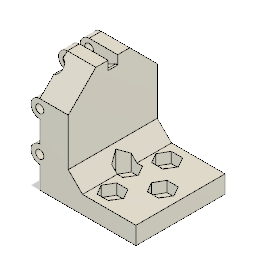
Anclaje base (Autodesk Fusion 360 design; units mm, degrees)
Autodesk Fusion 360 part; units mm, degrees
ref_plane "PlanoDeObra1" through (20, 0, 0) normal (1, 0, 0) x (0, 1, 0)
sketch "Boceto3" plane through (20, 0, 0) normal (1, 0, 0) x (0, 0, -1)
  line L0 (-0.475, 13.25) -> (-25.475, 13.25)
  line L1 (-25.475, 13.25) -> (-25.475, -16.75)
  line L2 (-25.475, -16.75) -> (-0.475, -16.75)
  line L3 (-0.475, -16.75) -> (-0.475, 13.25)
  line L4 (-25.475, -11.75) -> (-0.475, -11.75)
  line L5 (-17.2083, -5.5132) -> (-8.7417, -5.5132)
  line L6 (-8.7417, -5.5132) -> (-8.7417, -10.5132)
  line L7 (-8.7417, -10.5132) -> (-17.2083, -10.5132)
  line L8 (-17.2083, -10.5132) -> (-17.2083, -5.5132)
  line L9 (-3.9417, -5.5132) -> (-0.475, -5.5132)
  line L10 (-0.475, -5.5132) -> (-0.475, -10.5132)
  line L11 (-0.475, -10.5132) -> (-3.9417, -10.5132)
  line L12 (-3.9417, -10.5132) -> (-3.9417, -5.5132)
  line L13 (-22.0083, -5.5132) -> (-25.475, -5.5132)
  line L14 (-25.475, -5.5132) -> (-25.475, -10.5132)
  line L15 (-25.475, -10.5132) -> (-22.0083, -10.5132)
  line L16 (-22.0083, -10.5132) -> (-22.0083, -5.5132)
  line L17 (-19.5083, -9.4526) -> (-17.2083, -9.4526) construction
  line L18 (-8.7417, -8.7956) -> (-6.4417, -8.7956) construction
  line L19 (-22.0083, -5.5132) -> (-17.2083, -5.5132)
  line L20 (-17.2083, -10.5132) -> (-22.0083, -10.5132)
  line L21 (-8.7417, -5.5132) -> (-3.9417, -5.5132)
  line L22 (-3.9417, -10.5132) -> (-8.7417, -10.5132)
  line L23 (-0.475, -8.0132) -> (-25.475, -8.0132)
  line L24 (-25.475, 5.5132) -> (-22.0083, 5.5132)
  line L25 (-22.0083, 5.5132) -> (-22.0083, 0.5132)
  line L26 (-22.0083, 0.5132) -> (-25.475, 0.5132)
  line L27 (-25.475, 0.5132) -> (-25.475, 5.5132)
  line L28 (-3.9417, 5.5132) -> (-0.475, 5.5132)
  line L29 (-0.475, 5.5132) -> (-0.475, 0.5132)
  line L30 (-0.475, 0.5132) -> (-3.9417, 0.5132)
  line L31 (-3.9417, 0.5132) -> (-3.9417, 5.5132)
  line L32 (-22.0083, 5.5132) -> (-17.2083, 5.5132)
  line L33 (-17.2083, 5.5132) -> (-17.2083, 0.5132)
  line L34 (-17.2083, 0.5132) -> (-22.0083, 0.5132)
  line L35 (-3.9417, 5.5132) -> (-8.7417, 5.5132)
  line L36 (-8.7417, 5.5132) -> (-8.7417, 0.5132)
  line L37 (-8.7417, 0.5132) -> (-3.9417, 0.5132)
  line L38 (-25.475, 3.0132) -> (-0.475, 3.0132)
  line L39 (-17.7382, 13.25) -> (-25.475, 5.5132)
  line L40 (-8.2118, 13.25) -> (-0.475, 5.5132)
  line L41 (-19.5083, -5.5132) -> (-22.975, -5.5132) construction
  line L42 (-22.975, -10.5132) -> (-22.975, -5.5132) construction
  line L43 (-22.975, -10.5132) -> (-19.5083, -10.5132) construction
  line L44 (-19.5083, -10.5132) -> (-19.5083, -5.5132) construction
  line L45 (-2.975, -5.5132) -> (-6.4417, -5.5132) construction
  line L46 (-6.4417, -10.5132) -> (-6.4417, -5.5132) construction
  line L47 (-6.4417, -10.5132) -> (-2.975, -10.5132) construction
  line L48 (-2.975, -10.5132) -> (-2.975, -5.5132) construction
  line L49 (-2.975, 10.5132) -> (-6.4417, 10.5132) construction
  line L50 (-6.4417, 5.5132) -> (-6.4417, 10.5132) construction
  line L51 (-6.4417, 5.5132) -> (-2.975, 5.5132) construction
  line L52 (-2.975, 5.5132) -> (-2.975, 10.5132) construction
  line L53 (-19.5083, 10.5132) -> (-22.975, 10.5132) construction
  line L54 (-22.975, 5.5132) -> (-22.975, 10.5132) construction
  line L55 (-22.975, 5.5132) -> (-19.5083, 5.5132) construction
  line L56 (-19.5083, 5.5132) -> (-19.5083, 10.5132) construction
  line L57 (-11.2417, 10.5132) -> (-14.7083, 10.5132) construction
  line L58 (-14.7083, 5.5132) -> (-14.7083, 10.5132) construction
  line L59 (-14.7083, 5.5132) -> (-11.2417, 5.5132) construction
  line L60 (-11.2417, 5.5132) -> (-11.2417, 10.5132) construction
  line L61 (-14.7083, 5.5132) -> (-19.5083, 5.5132) construction
  line L62 (-6.4417, 5.5132) -> (-11.2417, 5.5132) construction
  line L63 (-22.0083, 0.5132) -> (-22.0083, -1.2368)
  line L64 (-22.0083, -1.2368) -> (-17.2083, -1.2368)
  line L65 (-17.2083, -1.2368) -> (-17.2083, 0.5132)
  line L66 (-8.7417, 0.5132) -> (-8.7417, -1.2368)
  line L67 (-8.7417, -1.2368) -> (-3.9417, -1.2368)
  line L68 (-3.9417, -1.2368) -> (-3.9417, 0.5132)
  line L69 (-22.0083, -5.5132) -> (-22.0083, -3.7632)
  line L70 (-22.0083, -3.7632) -> (-17.2083, -3.7632)
  line L71 (-17.2083, -3.7632) -> (-17.2083, -5.5132)
  line L72 (-3.9417, -5.5132) -> (-3.9417, -3.7632)
  line L73 (-3.9417, -3.7632) -> (-8.7417, -3.7632)
  line L74 (-8.7417, -3.7632) -> (-8.7417, -5.5132)
  line L75 (-8.7417, 0.5132) -> (-17.2083, 0.5132)
  line L76 (-17.2083, 5.5132) -> (-8.7417, 5.5132)
  line L77 (-8.2118, 13.25) -> (-8.2118, 8.25)
  line L78 (-8.2118, 8.25) -> (-17.7382, 8.25)
  line L79 (-17.7382, 8.25) -> (-17.7382, 13.25)
  line L80 (-8.2118, 10.75) -> (-17.7382, 10.75)
  line L81 (-14.325, 13.25) -> (-14.325, 8.25)
  line L82 (-11.625, 8.25) -> (-11.625, 13.25)
  line L83 (-11.625, 11.8923) -> (-8.2118, 11.8923) construction
  line L84 (-14.325, 11.8923) -> (-17.7382, 11.8923) construction
  line L85 (-11.625, 8.25) -> (-11.625, 7.5)
  line L86 (-11.625, 7.5) -> (-14.325, 7.5)
  line L87 (-14.325, 7.5) -> (-14.325, 8.25)
  line L88 (-17.2083, 5.0132) -> (-8.7417, 5.0132)
  line L89 (-17.2083, -3.7632) -> (-17.2083, -3.3632)
  line L90 (-17.2083, -3.3632) -> (-22.0083, -3.3632)
  line L91 (-22.0083, -3.3632) -> (-22.0083, -3.7632)
  line L92 (-3.9417, -3.7632) -> (-3.9417, -3.3632)
  line L93 (-3.9417, -3.3632) -> (-8.7417, -3.3632)
  line L94 (-8.7417, -3.3632) -> (-8.7417, -3.7632)
  line L95 (-3.9417, -1.2368) -> (-3.9417, -1.6368)
  line L96 (-3.9417, -1.6368) -> (-8.7417, -1.6368)
  line L97 (-8.7417, -1.6368) -> (-8.7417, -1.2368)
  line L98 (-17.2083, -1.2368) -> (-17.2083, -1.6368)
  line L99 (-17.2083, -1.6368) -> (-22.0083, -1.6368)
  line L100 (-22.0083, -1.6368) -> (-22.0083, -1.2368)
  line L101 (-8.7417, -6.0132) -> (-17.2083, -6.0132)
  dimension "d7" = 12
  dimension "d15" = 30
  dimension "d16" = 25
  dimension "d17" = 5
  dimension "d97" = 0.4
  dimension "d107" = 4.8
  dimension "d108" = 4.8
  dimension "d112" = 45
  dimension "d113" = 45
  dimension "d114" = 2.7
  dimension "d131" = 3.25
  dimension "d166" = 0.5
  dimension "d179" = 0.4
  dimension "d180" = 4.25
  dimension "d181" = 0.4
  dimension "d182" = 4.25
  dimension "d183" = 0.4
  dimension "d184" = 0.4
  dimension "d185" = 4.25
  dimension "d186" = 4.25
  dimension "d187" = 0.5
  constraint vertical L1
  constraint horizontal L2
  constraint vertical L3
  constraint coincident L1 L4.start
  constraint coincident L3 L4.end
  constraint perpendicular L3 L4
  constraint horizontal L5
  constraint vertical L6
  constraint horizontal L7
  constraint vertical L8
  constraint horizontal L9
  constraint vertical L10
  constraint horizontal L11
  constraint vertical L12
  constraint horizontal L13
  constraint vertical L14
  constraint horizontal L15
  constraint vertical L16
  constraint collinear L5 L13
  constraint collinear L5 L9
  constraint collinear L1 L14
  constraint collinear L3 L10
  constraint equal L17 L18
  constraint midpoint L10 L23.start
  constraint midpoint L14 L23.end
  constraint horizontal L24
  constraint vertical L25
  constraint horizontal L26
  constraint vertical L27
  constraint horizontal L28
  constraint vertical L29
  constraint horizontal L30
  constraint vertical L31
  constraint collinear L26 L30
  constraint collinear L1 L27
  constraint collinear L3 L29
  constraint horizontal L32
  constraint vertical L33
  constraint horizontal L34
  constraint horizontal L35
  constraint vertical L36
  constraint horizontal L37
  constraint midpoint L27 L38.start
  constraint midpoint L29 L38.end
  constraint coincident L0 L39.start
  constraint coincident L0 L40.start
  constraint equal L15 L43
  constraint equal L11 L47
  constraint equal L8 L44
  constraint equal L16 L44
  constraint coincident L8 L17.end
  constraint coincident L17.start L44
  constraint perpendicular L17 L44
  constraint coincident L6 L18.start
  constraint coincident L18.end L46
  constraint equal L12 L46
  constraint collinear L7 L47
  constraint equal L31 L50
  constraint equal L25 L56
  constraint coincident L30.end L31.start
  constraint coincident L25.end L26.start
  constraint equal L28 L49
  constraint equal L24 L53
  constraint collinear L28 L59
  constraint equal L34 L61
  constraint equal L37 L62
  constraint perpendicular L34 L63
  constraint perpendicular L25 L64
  constraint perpendicular L37 L66
  constraint perpendicular L36 L67
  constraint perpendicular L67 L68
  constraint perpendicular L64 L65
  constraint perpendicular L13 L69
  constraint perpendicular L16 L70
  constraint perpendicular L21 L72
  constraint perpendicular L72 L73
  constraint perpendicular L73 L74
  constraint perpendicular L70 L71
  constraint perpendicular L18 L46
  constraint perpendicular L0 L77
  constraint perpendicular L77 L78
  constraint perpendicular L78 L79
  constraint equal L58 L79
  constraint midpoint L77 L80.start
  constraint midpoint L79 L80.end
  constraint parallel L79 L81
  constraint parallel L77 L82
  constraint coincident L82 L83.start
  constraint coincident L77 L83.end
  constraint perpendicular L77 L83
  constraint coincident L81 L84.start
  constraint coincident L79 L84.end
  constraint perpendicular L79 L84
  constraint equal L83 L84
  constraint perpendicular L78 L85
  constraint perpendicular L78 L87
  constraint parallel L78 L86
  constraint coincident L33 L88.start
  constraint coincident L36 L88.end
  constraint perpendicular L36 L88
  constraint perpendicular L70 L89
  constraint perpendicular L71 L90
  constraint perpendicular L90 L91
  constraint perpendicular L73 L92
  constraint perpendicular L72 L93
  constraint perpendicular L93 L94
  constraint perpendicular L67 L95
  constraint perpendicular L95 L96
  constraint perpendicular L96 L97
  constraint perpendicular L64 L98
  constraint perpendicular L65 L99
  constraint perpendicular L99 L100
  constraint coincident L6 L101.start
  constraint coincident L8 L101.end
  constraint perpendicular L8 L101
  measures "d15" distance of L0.end L1.end
  measures "d16" distance of L1.end L2.end
  measures "d17" distance of L2 L4
  measures "d107" distance of L6 L12
  measures "d108" distance of L31 L36
  measures "d112" angle of L28.end L40.start L50.start
  measures "d113" angle of L24.start L39.start L55.end
  measures "d114" distance of L81 L82
  measures "d131" distance of L80 L86
  measures "d166" distance of L76 L88
  measures "d179" distance of L70 L90
  measures "d180" distance of L23 L70
  measures "d181" distance of L73 L93
  measures "d182" distance of L23 L73
  measures "d183" distance of L67 L96
  measures "d184" distance of L64 L99
  measures "d185" distance of L38 L64
  measures "d186" distance of L38 L67
  measures "d187" distance of L5 L101
extrude "Extruir5" add sketch "Boceto3" along normal blind 8 contours L0 L77 L80 L82 | L24 L28 L32 L35 L39 L40 L76 L77 L78 L79 L85 L86 L87 | L3 L28 L29 L31 L38 | L0 L80 L81 L82 | L77 L78 L80 L82 | L3 L29 L30 L31 L38 | L31 L35 L36 L38 | L0 L79 L80 L81 | L78 L80 L81 L82 | L1 L3 L5 L9 L13 L26 L30 L63 L65 L66 L68 L69 L71 L72 L74 L75 L89 L90 L91 L92 L93 L94 L95 L96 L97 L98 L99 L100 | L31 L36 L37 L38 | L33 L36 L76 L88 | L78 L79 L80 L81 | L78 L85 L86 L87 | L3 L9 L10 L12 L23 | L37 L66 L67 L68 | L33 L36 L38 L88 | L33 L36 L38 L75 | L25 L32 L33 L38 | L1 L24 L25 L27 L38 | L3 L10 L11 L12 L23 | L6 L12 L21 L23 | L21 L72 L73 L74 | L67 L95 L96 L97 | L25 L33 L34 L38 | L1 L25 L26 L27 L38 | L1 L3 L4 L7 L11 L15 L20 L22 | L6 L12 L22 L23 | L5 L6 L8 L101 | L73 L92 L93 L94 | L34 L63 L64 L65 | L1 L2 L3 L4 | L6 L8 L23 L101 | L6 L7 L8 L23 | L8 L16 L19 L23 | L19 L69 L70 L71 | L64 L98 L99 L100 | L1 L13 L14 L16 L23 | L8 L16 L20 L23 | L70 L89 L90 L91 | L1 L14 L15 L16 L23
extrude "Extruir6" add sketch "Boceto3" along normal blind 27 contours L1 L2 L3 L4
revolve "Revolución13" add sketch "Boceto3" angle 360 about axis through (20, -8.0132, 0.475) along (0, 0, 1) contours L3 L9 L10 L12 L23 | L6 L8 L23 L101 | L1 L13 L14 L16 L23
revolve "Revolución14" cut sketch "Boceto3" angle 360 about axis through (20, -8.0132, 0.475) along (0, 0, 1) contours L6 L12 L21 L23 | L21 L72 L73 L74 | L73 L92 L93 L94 | L8 L16 L19 L23 | L19 L69 L70 L71 | L70 L89 L90 L91
revolve "Revolución15" add sketch "Boceto3" angle 360 about axis through (20, 3.0132, 25.475) along (0, 0, -1) contours L3 L28 L29 L31 L38 | L33 L36 L38 L88 | L1 L24 L25 L27 L38
revolve "Revolución16" cut sketch "Boceto3" angle 360 about axis through (20, 3.0132, 25.475) along (0, 0, -1) contours L31 L36 L37 L38 | L37 L66 L67 L68 | L67 L95 L96 L97 | L25 L33 L34 L38 | L34 L63 L64 L65 | L64 L98 L99 L100
revolve "Revolución19" add sketch "Boceto3" angle 360 about axis through (20, 10.75, 8.2118) along (0, 0, 1) contours L0 L77 L80 L82 | L0 L79 L80 L81
revolve "Revolución20" cut sketch "Boceto3" angle 360 about axis through (20, 10.75, 8.2118) along (0, 0, 1) contours L78 L80 L81 L82 | L78 L85 L86 L87
extrude "Extruir9" cut sketch "Boceto3" along normal blind 10 contours L0 L80 L81 L82
hole "Agujero7" at (20, 3.0132, 25.475) direction (0, 0, -1) diameter 2.3 depth 30 tip angle 118
hole "Agujero8" at (20, -8.0132, 25.475) direction (0, 0, -1) diameter 2.3 depth 30 tip angle 118
hole "Agujero11" at (20, 10.75, 17.7382) direction (0, 0, -1) diameter 2.5 depth 14 tip angle 118
hole "Agujero12" at (20, 10.75, 8.2118) direction (0, 0, 1) diameter 2.5 depth 14 tip angle 118
ref_plane "PlanoDeObra2" through (37.5, -11.75, 12.975) normal (0, 1, 0) x (0, 0, 1)
sketch "Boceto4" plane through (37.5, -11.75, 12.975) normal (0, 1, 0) x (1, 0, 0)
  circle A0 centre (4.5, -3) radius 1.2645 construction
  arc A1 (-6.5, -3.7739) -> (-6.5, -2.2261) centre (-5.5, -3) ccw construction
  circle A2 centre (-1.9279, 4.6604) radius 1.2645 construction
  line L0 (-9.5, 12.5) -> (-9.5, -12.5)
  line L1 (-9.5, -12.5) -> (9.5, -12.5)
  line L2 (9.5, -12.5) -> (9.5, 12.5)
  line L3 (9.5, 12.5) -> (-9.5, 12.5)
  line L4 (9.5, 0) -> (-9.5, 0) construction
  line L5 (4.5, -3) -> (-5.5, -3) construction
  line L6 (-1.9279, 4.6604) -> (4.5, -3) construction
  line L7 (-5.5, -3) -> (-5.5, 0) construction
  circle A3 centre (-5.5, 0) radius 1.2645
  line L8 (4.5, -3) -> (4.5, 0) construction
  circle A4 centre (4.5, 0) radius 1.2645
  line L9 (4.5, 0) -> (-1.9279, 7.6604) construction
  circle A5 centre (-1.9279, 7.6604) radius 1.2645
  circle A6 centre (-1.9279, -7.6604) radius 1.2645
  dimension "d85" = 10
  dimension "d87" = 10
  dimension "d88" = 50
  dimension "d89" = 10
  dimension "d90" = 50
  constraint midpoint L2 L4.start
  constraint midpoint L0 L4.end
  constraint coincident A0.centre L5.start
  constraint coincident A1.centre L5.end
  constraint coincident A2.centre L6.start
  constraint coincident L4 L7.end
  constraint perpendicular L4 L7
  constraint coincident L7.end A3.centre
  constraint equal A1 A3
  constraint coincident L4 L8.end
  constraint perpendicular L4 L8
  constraint coincident L8.end A4.centre
  constraint equal A0 A4
  constraint coincident L9.end A5.centre
  constraint equal A2 A5
  constraint symmetric L4 A5 A6
  measures "d85" distance of A0.centre A1.centre
  measures "d87" distance of A2.centre A0.centre
  measures "d88" angle of A0.centre A1.centre A2.centre
  measures "d89" distance of L8.end L9.end
  measures "d90" angle of L7.end L8.end L9.end
extrude "Extruir8" cut sketch "Boceto4" against normal blind 10 contours A3 | A4 | A5 | A6
ref_plane "PlanoDeObra3" through (22.75, 10.375, 12.625) normal (0, 0, 1) x (1, 0, 0)
sketch "Boceto5" plane through (22.75, 10.375, 11.625) normal (0, 0, 1) x (1, 0, 0)
  arc A0 (-2.75, -2.875) -> (0.5, 0.375) centre (-2.75, 0.375) ccw construction
  line L0 (0.5, 0.375) -> (5.25, 0.375) construction
  circle A1 centre (-2.75, 0.375) radius 1.25 construction
  line L1 (-2.75, -2.875) -> (-2.75, -4.8618) construction
  line L2 (-5.2247, -4.1459) -> (-1.8318, -0.4732)
  line L3 (-3.7556, -5.503) -> (3.0301, 1.8423)
  line L4 (1.561, 3.1995) -> (3.0301, 1.8423)
  line L5 (-3.7556, -5.503) -> (-5.2247, -4.1459)
  line L6 (-1.8318, -0.4732) -> (1.561, 3.1995)
  arc A2 (-2.75, -5.3618) -> (-2.75, -9.3618) centre (-2.75, -7.3618) ccw
  dimension "d133" = 2
  dimension "d134" = 2
  dimension "d135" = 10
  constraint coincident A0.start L1.start
  constraint parallel L2 L3
  constraint tangent A1 L2
  constraint perpendicular L2 L4
  constraint coincident A1 L2.end
  constraint parallel L3 L6
  constraint equal L2 L6
  constraint tangent L3 A2
  measures "d133" distance of A0 A1
  measures "d134" distance of L2 L3
  measures "d135" distance of L4 L5
extrude "Extruir10" cut sketch "Boceto5" along normal up to surface (2.7 mm away)
chamfer "Chaflán3" distance 3 angle 55 1 edges at (24.4246, 10.75, 12.975) measured on face at (25.6164, 10.75, 12.525)
chamfer "Chaflán5" distance 4 angle 45 1 edges at (28, -11.75, 12.975)
sketch "Boceto7" plane through (0, -11.75, 0) normal (0, 1, 0) x (-1, 0, 0)
  line L0 (-32, 0.475) -> (-32, 11.7105)
  arc A0 (-32, 14.2395) -> (-32, 11.7105) centre (-32, 12.975) ccw
  line L1 (-32, 14.2395) -> (-32, 25.475)
  line L2 (-32, 25.475) -> (-47, 25.475)
  line L3 (-47, 25.475) -> (-47, 0.475)
  line L4 (-47, 0.475) -> (-32, 0.475)
  circle A1 centre (-35.5721, 20.6354) radius 1.2645
  circle A2 centre (-42, 12.975) radius 1.2645
  circle A3 centre (-35.5721, 5.3146) radius 1.2645
  circle A4 centre (-42, 12.975) radius 1.2645
  circle A5 centre (-35.5721, 20.6354) radius 1.2645
  circle A6 centre (-35.5721, 5.3146) radius 1.2645
  arc A7 (-32, 14.2395) -> (-32, 11.7105) centre (-32, 12.975) ccw
  line L5 (-40.4123, 10.225) -> (-43.5877, 10.225)
  line L6 (-45.1754, 12.975) -> (-43.5877, 10.225)
  line L7 (-45.1754, 12.975) -> (-43.5877, 15.725)
  line L8 (-43.5877, 15.725) -> (-40.4123, 15.725)
  line L9 (-40.4123, 15.725) -> (-38.8246, 12.975)
  line L10 (-38.8246, 12.975) -> (-40.4123, 10.225)
  line L11 (-38.8246, 12.975) -> (-45.1754, 12.975) construction
  line L12 (-43.5877, 10.225) -> (-40.4123, 15.725) construction
  line L13 (-40.4123, 10.225) -> (-43.5877, 15.725) construction
  line L14 (-33.9844, 8.0646) -> (-37.1598, 2.5646) construction
  line L15 (-32.3967, 5.3146) -> (-38.7476, 5.3146) construction
  line L16 (-33.9844, 2.5646) -> (-37.1598, 8.0646) construction
  line L17 (-33.9844, 2.5646) -> (-37.1598, 2.5646)
  line L18 (-37.1598, 2.5646) -> (-38.7476, 5.3146)
  line L19 (-38.7476, 5.3146) -> (-37.1598, 8.0646)
  line L20 (-37.1598, 8.0646) -> (-33.9844, 8.0646)
  line L21 (-33.9844, 8.0646) -> (-32.3967, 5.3146)
  line L22 (-32.3967, 5.3146) -> (-33.9844, 2.5646)
  line L23 (-32.3967, 20.6354) -> (-38.7476, 20.6354) construction
  line L24 (-33.9844, 17.8854) -> (-37.1598, 23.3854) construction
  line L25 (-37.1598, 17.8854) -> (-33.9844, 23.3854) construction
  line L26 (-33.9844, 17.8854) -> (-37.1598, 17.8854)
  line L27 (-37.1598, 17.8854) -> (-38.7476, 20.6354)
  line L28 (-38.7476, 20.6354) -> (-37.1598, 23.3854)
  line L29 (-37.1598, 23.3854) -> (-33.9844, 23.3854)
  line L30 (-33.9844, 23.3854) -> (-32.3967, 20.6354)
  line L31 (-32.3967, 20.6354) -> (-33.9844, 17.8854)
  line L32 (-30.4123, 15.725) -> (-33.5877, 10.225) construction
  line L33 (-30.4123, 10.225) -> (-33.5877, 15.725) construction
  line L34 (-35.1754, 12.975) -> (-28.8246, 12.975) construction
  line L35 (-30.4123, 10.225) -> (-33.5877, 10.225)
  line L36 (-35.1754, 12.975) -> (-33.5877, 10.225)
  line L37 (-33.5877, 15.725) -> (-35.1754, 12.975)
  line L38 (-30.4123, 15.725) -> (-33.5877, 15.725)
  line L39 (-28.8246, 12.975) -> (-30.4123, 15.725)
  line L40 (-30.4123, 10.225) -> (-28.8246, 12.975)
  circle A8 centre (-32, 12.975) radius 1.2645
  dimension "d150" = 5.5
  dimension "d151" = 60
  dimension "d152" = 60
  dimension "d153" = 60
  dimension "d154" = 60
  dimension "d155" = 5.5
  dimension "d156" = 60
  dimension "d157" = 60
  dimension "d158" = 5.5
  dimension "d159" = 60
  dimension "d160" = 60
  dimension "d161" = 5.5
  constraint midpoint A2.centre L13
  constraint midpoint L11 L13
  constraint equal L12 L13
  constraint equal L11 L12
  constraint midpoint L12 L13
  constraint horizontal L5
  constraint midpoint A3.centre L14
  constraint midpoint L14 L16
  constraint midpoint A3.centre L15
  constraint equal L14 L16
  constraint equal L14 L15
  constraint horizontal L17
  constraint midpoint A1.centre L25
  constraint midpoint A1.centre L24
  constraint midpoint A1.centre L23
  constraint equal L24 L25
  constraint equal L23 L25
  constraint horizontal L26
  constraint midpoint A0.centre L32
  constraint midpoint A0.centre L33
  constraint midpoint A0.centre L34
  constraint equal L32 L33
  constraint equal L32 L34
  constraint horizontal L35
  constraint concentric A7 A8
  constraint coincident L0.end A8
  measures "d150" distance of L5 L8
  measures "d151" angle of L12 L13
  measures "d152" angle of L11 L13
  measures "d153" angle of L14 L16
  measures "d154" angle of L15 L16
  measures "d155" distance of L17 L20
  measures "d156" angle of L24 L25
  measures "d157" angle of L23 L24
  measures "d158" distance of L26 L29
  measures "d159" angle of L32 L33
  measures "d160" angle of L33 L34
  measures "d161" distance of L35 L38
extrude "Extruir11" cut sketch "Boceto7" along normal blind -3 and the other way blind -5 contours L0 A0 L1 A7 L35 L36 L37 L38 A8 | L0 L1 L35 L38 L39 L40 A8 | L5 L6 L7 L8 L9 L10 | L17 L18 L19 L20 L21 L22 | L26 L27 L28 L29 L30 L31
hole "Agujero13" at (35.5721, -14.75, 5.3146) direction (0, -1, 0) diameter 3 depth 3 tip angle 118
hole "Agujero14" at (42, -14.75, 12.975) direction (0, -1, 0) diameter 3 depth 3 tip angle 118
hole "Agujero15" at (32, -14.75, 12.975) direction (0, -1, 0) diameter 3 depth 3 tip angle 118
hole "Agujero16" at (35.5721, -14.75, 20.6354) direction (0, -1, 0) diameter 3 depth 3 tip angle 118
fillet "Empalme5" radius 1.5 1 edges at (20, 5.9605, 12.975)
move_face "CarasDesfase1" offset -0.2 1 faces at (20.7712, 6.7953, 13.425)
equation "d89 = d87"
equation "d90 = d88"
equation "d107 = d108"
equation "d131 = 2 mm + ( 2.5 / 2 ) * 1 mm"
equation "d155 = d150"
equation "d158 = d150"
equation "d161 = d150"
equation "d181 = d179"
equation "d182 = d180"
equation "d183 = d181"
equation "d184 = d179"
equation "d185 = d180"
equation "d186 = d180"
equation "d187 = d166"
